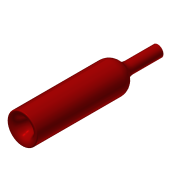
# Autodesk Inventor part: WINE_RED_1
Saved by Autodesk Inventor 2018 (Build 220112000, 112)
## iProperties
Created: 2014-03-10
Part Number: WINE_RED_1
Material: Plaster
Document SubType Name: Modeling
Designer: Zarko G.
Mass: 740.758 g
Surface Area: 509.269 cm^2
Volume: 661.392 cm^3
Density: 1.12 g/cm^3
Appearance: Smooth - Red
Author: Zarko G.
Autodesk Inventor part; units mm, degrees
ref_plane "YZ Plane" through (0, 0, 0) normal (1, 0, 0) x (0, 1, 0)
ref_plane "XZ Plane" through (0, 0, 0) normal (0, 1, 0) x (-1, 0, 0)
ref_plane "XY Plane" through (0, 0, 0) normal (0, 0, 1) x (1, 0, 0)
sketch "Sketch1" plane through (0, 0, 0) normal (0, 0, 1) x (1, 0, 0)
  spline S0 degree 3 poles (29.6986, 3.3634) (29.8814, 3.3355) (30.0671, 3.3331) (30.434, 3.3795) (30.6134, 3.428) (31.0231, 3.6024) (31.2405, 3.7503) (31.6064, 4.121) (31.7514, 4.3403) (31.9491, 4.8222) (32, 5.0801) (32, 5.3405) knots -0.34533 -0.34533 -0.34533 -0.34533 -0.289859 -0.289859 -0.234387 -0.234387 -0.156258 -0.156258 -0.078129 -0.078129 0 0 0 0 construction
  line L0 (32, 5.3405) -> (32, 190) construction
  arc A0 (32, 190) -> (20.7559, 211.9261) centre (5, 190) ccw construction
  arc A1 (12, 229) -> (20.7559, 211.9261) centre (33.025, 229) ccw construction
  line L1 (12, 229) -> (12, 300) construction
  line L2 (12, 300) -> (14, 300) construction
  arc A2 (15, 299) -> (14, 300) centre (14, 299) ccw construction
  line L3 (15, 299) -> (15, 229) construction
  arc A3 (15, 229) -> (22.5065, 214.3623) centre (33.025, 229) ccw construction
  arc A4 (35, 190) -> (22.5065, 214.3623) centre (5, 190) ccw construction
  line L4 (35, 190) -> (35, 5.3405) construction
  spline S1 degree 3 poles (35, 5.3405) (35, 4.8783) (34.9359, 4.4182) (34.6831, 3.5289) (34.4957, 3.1039) (33.9101, 2.157) (33.4628, 1.6755) (32.4088, 0.9109) (31.8121, 0.6352) (30.5467, 0.3281) (29.89, 0.2995) (29.2464, 0.3977) knots -0.863326 -0.863326 -0.863326 -0.863326 -0.724646 -0.724646 -0.585967 -0.585967 -0.390644 -0.390644 -0.195322 -0.195322 0 0 0 0 construction
  spline S2 degree 3 poles (29.2464, 0.3977) (26.1774, 0.8656) (23.7647, 1.729) (20.1854, 3.8713) (18.825, 5.0891) (16.2221, 8.372) (15.193, 10.3823) (12.8144, 15.5018) (11.5745, 18.6403) (8.5374, 22.145) (7.4227, 23.0499) (5.2311, 24.1468) (4.3215, 24.4544) (2.2754, 24.9009) (1.1405, 24.9993) (0.0085, 25) (0.0043, 25) (0, 25) knots -3.773071 -3.773071 -3.773071 -3.773071 -3.15254 -3.15254 -2.633774 -2.633774 -2.013412 -2.013412 -1.072391 -1.072391 -0.62775 -0.62775 -0.338334 -0.338334 0 0 0.001276 0.001276 0.001276 0.001276 construction
  spline S3 degree 3 poles (0, 25) (-0.0043, 25) (-0.0085, 25) (-1.1405, 24.9993) (-2.2754, 24.9009) (-4.3215, 24.4544) (-5.2311, 24.1468) (-7.4227, 23.0499) (-8.5374, 22.145) (-11.5745, 18.6403) (-12.8144, 15.5018) (-15.193, 10.3823) (-16.2221, 8.372) (-18.825, 5.0891) (-20.1854, 3.8713) (-23.7647, 1.729) (-26.1774, 0.8656) (-29.2464, 0.3977) knots -5.664841 -5.664841 -5.664841 -5.664841 -5.662926 -5.662926 -5.155127 -5.155127 -4.720749 -4.720749 -4.053395 -4.053395 -2.641037 -2.641037 -1.709948 -1.709948 -0.931342 -0.931342 0 0 0 0 construction
  spline S4 degree 3 poles (-29.2464, 0.3977) (-29.7034, 0.328) (-30.1678, 0.322) (-31.0851, 0.4379) (-31.5335, 0.5591) (-32.5578, 0.9953) (-33.1013, 1.3649) (-34.016, 2.2917) (-34.3785, 2.84) (-34.8728, 4.0446) (-35, 4.6895) (-35, 5.3405) knots -0.863326 -0.863326 -0.863326 -0.863326 -0.724646 -0.724646 -0.585967 -0.585967 -0.390644 -0.390644 -0.195322 -0.195322 0 0 0 0 construction
  line L5 (-35, 5.3405) -> (-35, 190) construction
  arc A5 (-22.5065, 214.3623) -> (-35, 190) centre (-5, 190) ccw construction
  arc A6 (-22.5065, 214.3623) -> (-15, 229) centre (-33.025, 229) ccw construction
  line L6 (-15, 229) -> (-15, 299) construction
  arc A7 (-14, 300) -> (-15, 299) centre (-14, 299) ccw construction
  line L7 (-14, 300) -> (-12, 300) construction
  line L8 (-12, 291.9261) -> (-12, 229) construction
  arc A8 (-20.7559, 211.9261) -> (-12, 229) centre (-33.025, 229) ccw
  arc A9 (-20.7559, 211.9261) -> (-32, 190) centre (-5, 190) ccw
  line L9 (-32, 190) -> (-32, 5.3405)
  spline S5 degree 3 poles (-32, 5.3405) (-32, 5.1556) (-31.9744, 4.9716) (-31.8733, 4.6159) (-31.7983, 4.4459) (-31.5641, 4.0671) (-31.3851, 3.8745) (-30.9635, 3.5687) (-30.7248, 3.4584) (-30.2187, 3.3356) (-29.956, 3.3241) (-29.6986, 3.3634) knots -0.34533 -0.34533 -0.34533 -0.34533 -0.289859 -0.289859 -0.234387 -0.234387 -0.156258 -0.156258 -0.078129 -0.078129 0 0 0 0
  spline S6 degree 3 poles (-29.6986, 3.3634) (-26.8246, 3.8016) (-24.8387, 4.5825) (-22.0363, 6.2598) (-20.9487, 7.2392) (-18.7688, 9.9887) (-17.8486, 11.7864) (-15.5028, 16.8354) (-14.1571, 20.2412) (-10.6891, 24.2428) (-9.2888, 25.4707) (-6.3501, 26.9415) (-5.2055, 27.3322) (-2.7032, 27.8781) (-1.3582, 27.9992) (-0.0091, 28) (-0.0046, 28) (0, 28) knots -4.912754 -4.912754 -4.912754 -4.912754 -4.195659 -4.195659 -3.557464 -3.557464 -2.744003 -2.744003 -1.389042 -1.389042 -0.768144 -0.768144 -0.403356 -0.403356 0 0 0.00137 0.00137 0.00137 0.00137
  spline S7 degree 3 poles (0, 28) (0.0046, 28) (0.0091, 28) (1.3582, 27.9992) (2.7032, 27.8781) (5.2055, 27.3322) (6.3501, 26.9415) (9.2888, 25.4707) (10.6891, 24.2428) (14.1571, 20.2412) (15.5028, 16.8354) (17.8486, 11.7864) (18.7688, 9.9887) (20.9487, 7.2392) (22.0363, 6.2598) (24.8387, 4.5825) (26.8246, 3.8016) (29.6986, 3.3634) knots -5.976652 -5.976652 -5.976652 -5.976652 -5.974985 -5.974985 -5.484417 -5.484417 -5.040754 -5.040754 -4.285607 -4.285607 -2.637676 -2.637676 -1.64833 -1.64833 -0.872146 -0.872146 0 0 0 0 construction
  line L10 (0, 28) -> (0, 291.9261)
  line L11 (-12, 291.9261) -> (-12, 229)
  line L12 (11.5, 260) -> (-11.5, 260) construction
  line L13 (0, 291.9261) -> (-12, 291.9261)
  point P0 (0, 0)
  point P1 (0, 260)
  point P2 (-12, 260)
  dimension "d1" = 80
  constraints: 26 end point, 20 point on circle, 10 centre point, 8 vertical, 3 horizontal, 3 point on line, 1 collinear, 1 parallel, 1 tangent, 64 other
  measures "d1" distance from line of A8.start L13
revolve "Revolution1" add sketch "Sketch1" angle 360 about axis through (0, 28, 0) along (0, 1, 0)
body "Solid1"
